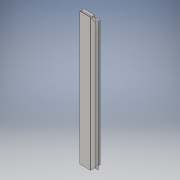
# Autodesk Inventor part: Cabinet Moulding Long
Saved by Autodesk Inventor 2016 (Build 200138000, 138)
## iProperties
Created: 2017-11-05
Part Number: Cabinet Moulding Long
Material: Wood (Oak)
Document SubType Name: Modeling
Designer: mathaetaes
Density: 0.76 g/cm^3
Appearance: White Oak - Natural Medium Gloss
Author: mathaetaes
Autodesk Inventor part; units mm, degrees
ref_plane "YZ Plane" through (0, 0, 0) normal (1, 0, 0) x (0, 1, 0)
ref_plane "XZ Plane" through (0, 0, 0) normal (0, 1, 0) x (-1, 0, 0)
ref_plane "XY Plane" through (0, 0, 0) normal (0, 0, 1) x (1, 0, 0)
sketch "Sketch1" plane through (0, 0, 0) normal (0, 1, 0) x (-1, 0, 0)
  line L0 (0, 0) -> (-32.8112, 0)
  line L1 (-38.1, -15.875) -> (0, -15.875)
  line L2 (0, -15.875) -> (0, 0)
  line L3 (0, -15.875) -> (-38.1, -15.875)
  line L4 (-38.1, -15.875) -> (-38.1, -10.5833)
  line L5 (0, -17.5053) -> (0, -15.875)
  line L6 (-28.575, -10.5833) -> (-28.575, -4.2333)
  line L7 (0, -12.2137) -> (0, -17.5053)
  line L8 (-28.575, -4.2333) -> (-38.1, -4.2333)
  line L9 (-38.1, -10.5833) -> (-38.1, -15.875)
  line L10 (-28.575, -10.5833) -> (-38.1, -10.5833)
  line L11 (0, 0) -> (-28.575, 0)
  line L12 (-28.575, 0) -> (-28.575, -0.7937)
  line L13 (-28.575, -0.7937) -> (0, -0.7937)
  line L14 (0, -0.7937) -> (0, 0)
  arc A0 (-28.575, -0.7937) -> (-38.1, -4.2333) centre (-28.575, -15.702) ccw
  dimension "d0" = 38.1
  dimension "d5" = 9.525
  dimension "d6" = 0.7937
  dimension "d10" = 9.525
  dimension "d11" = 28.575
  dimension "d13" = 15.875
  dimension "d14" = 14.9083
  dimension "d15" = 6.35
  constraints: 30 end point, 6 parallel, 4 horizontal, 4 perpendicular, 2 point on circle, 1 centre point, 1 collinear, 1 tangent
  measures "d0" distance of L1.end L1.start
  measures "d5" distance of L6.end L8.end
  measures "d6" distance of L11.end L12.end
  measures "d10" distance of L6.start L4.end
  measures "d11" distance of L0.start L11.end
  measures "d13" distance of L1.end L0.start
  measures "d14" radius of A0
  measures "d15" distance of L6.start L6.end
extrude "Extrusion1" add sketch "Sketch1" along normal blind 407.9875
sketch "Sketch2" plane through (0, 0, -15.875) normal (-1, 0, 0) x (0, 0, 1)
  line L0 (15.875, 0) -> (0, 0)
  line L1 (0, 0) -> (0, 38.1)
  line L2 (0, 38.1) -> (5.2897, 38.1)
  line L3 (5.2897, 28.575) -> (11.6397, 28.575)
  line L4 (11.6397, 28.575) -> (11.6397, 38.1)
  line L5 (5.2897, 28.575) -> (5.2897, 38.1)
  line L6 (15.875, 28.575) -> (15.0538, 28.575)
  line L7 (15.875, 0) -> (15.875, 28.575)
  arc A0 (15.0538, 28.575) -> (11.6397, 38.1) centre (0.1441, 28.6051) ccw
  line L8 (0, 407.9875) -> (0, 369.8875)
  line L9 (0, 369.8875) -> (5.3061, 369.8875)
  line L10 (5.3061, 369.8875) -> (5.3061, 379.4125)
  line L11 (5.3061, 379.4125) -> (11.6561, 379.4125)
  line L12 (11.6561, 379.4125) -> (11.6561, 369.8875)
  line L13 (15.0538, 379.4125) -> (15.875, 379.4125)
  line L14 (0, 407.9875) -> (15.875, 407.9875) projected
  line L15 (15.875, 379.4125) -> (15.875, 407.9875)
  line L16 (0, 407.9875) -> (15.875, 407.9875)
  arc A1 (11.6561, 369.8875) -> (15.0538, 379.4125) centre (0.1441, 379.3625) ccw
  dimension "d17" = 38.1
  dimension "d18" = 9.525
  dimension "d19" = 6.35
  dimension "d21" = 14.9098
  dimension "d22" = 14.9098
  constraints: 32 end point, 6 equal length, 5 vertical, 4 point on circle, 3 collinear, 3 perpendicular, 2 centre point, 2 horizontal, 1 parallel, 1 point on line
  measures "d17" distance of L0.end L1.end
  measures "d18" distance of L3.start L2.end
  measures "d19" distance of L3.start L3.end
  measures "d21" radius of A0
  measures "d22" radius of A1
extrude "Extrusion2" [suppressed]
equation "\"d5\" = d10"
body "Solid1"
